Stepper Motor Holder (Autodesk Fusion 360 design; units mm, degrees)
Autodesk Fusion 360 part; units mm, degrees
note: some values were not read from the file. Set by a fixed rule: which face or edge a step refers to.
sketch "Sketch1" plane through (0, 0, 0) normal (0, 0, 1) x (1, 0, 0)
  circle A0 centre (0, 0) radius 11
  circle A1 centre (-15.5, 15.5) radius 1.5
  circle A2 centre (15.5, 15.5) radius 1.5
  circle A3 centre (15.5, -15.5) radius 1.5
  circle A4 centre (-15.5, -15.5) radius 1.5
  line L0 (23.5, -23.5) -> (-23.5, -23.5)
  line L1 (-23.5, -23.5) -> (-23.5, 23.5)
  line L2 (-23.5, 23.5) -> (23.5, 23.5)
  line L3 (23.5, 23.5) -> (23.5, -23.5)
  line L4 (23.5, -23.5) -> (-23.5, 23.5) construction
  line L5 (-23.5, -23.5) -> (23.5, 23.5) construction
  dimension "d3" = 22
  dimension "d4" = 3
  dimension "d5" = 15.5
  dimension "d6" = 15.5
  dimension "d7" = 31
  dimension "d8" = 15.5
  dimension "d9" = 47
  dimension "d10" = 47
  constraint horizontal A1.centre A2.centre
  constraint vertical A2.centre A3.centre
  constraint horizontal A3.centre A4.centre
  constraint vertical A1.centre A4.centre
  constraint equal A1 A2
  constraint equal A1 A4
  constraint equal A3 A4
  constraint coincident A0.centre origin
  constraint horizontal L0
  constraint perpendicular L0 L1
  constraint parallel L0 L2
  constraint parallel L1 L3
  constraint coincident L4 A0.centre
  constraint coincident L5 A0.centre
  measures "d3" diameter of A0
  measures "d4" diameter of A2
  measures "d5" horizontal distance of A0.centre A3.centre
  measures "d6" horizontal distance of A0.centre A4.centre
  measures "d7" distance of A1.centre A4.centre
  measures "d8" vertical distance of A0.centre A4.centre
  measures "d9" distance of L1.end L2.end
  measures "d10" distance of L0.end L1.end
extrude "Extrude1" add sketch "Sketch1" along normal blind 2
sketch "Sketch2" plane through (-23.5, 0, 0) normal (-1, 0, 0) x (0, -1, 0)
  line L0 (-23.5, 0) -> (23.5, 0)
  line L1 (23.5, 0) -> (23.5, 2)
  line L2 (23.5, 2) -> (-23.5, 2)
  line L3 (-23.5, 2) -> (-23.5, 0)
  line L4 (23.5, 2) -> (23.5, 55)
  line L5 (21, 2) -> (21, 47.4468)
  line L6 (-23.5, 2) -> (-23.5, 55)
  line L7 (-23.5, 55) -> (23.5, 55)
  line L8 (21, 47.4468) -> (21, 55)
  line L9 (23.5, 4.5) -> (-23.5, 4.5)
  line L10 (-21, 2) -> (-21, 55)
  dimension "d13" = 53
  dimension "d14" = 2.5
  dimension "d64" = 2.5
  dimension "d65" = 2.5
  dimension "d154" = 42
  constraint coincident L1.end L2.start
  constraint perpendicular L2 L4
  constraint coincident L2 L5.start
  constraint perpendicular L2 L5
  constraint coincident L2.end L3.start
  constraint perpendicular L2 L6
  constraint perpendicular L4 L7
  constraint coincident L7 L8.end
  constraint perpendicular L7 L8
  constraint coincident L4 L9.start
  constraint coincident L6 L9.end
  constraint perpendicular L6 L9
  constraint coincident L2 L10.start
  constraint coincident L7 L10.end
  constraint perpendicular L7 L10
  measures "d13" distance of L1.end L4.end
  measures "d14" distance of L4 L5
  measures "d64" distance of L2 L9
  measures "d65" distance of L6 L10
  measures "d154" distance of L5 L10
extrude "Extrude2" add sketch "Sketch2" against normal blind 2.45 contours L2 L6 L9 L10 | L2 L4 L5 L9 | L2 L5 L9 L10 | L6 L7 L9 L10 | L4 L5 L7 L8 L9 | L5 L7 L8 L9 L10
extrude "Extrude4" add sketch "Sketch2" along normal blind 2.45 from surface at -47 contours L2 L6 L9 L10 | L2 L4 L5 L9 | L2 L5 L9 L10 | L6 L7 L9 L10 | L4 L5 L7 L8 L9 | L5 L7 L8 L9 L10
extrude "Extrude5" add sketch "Sketch2" against normal up to surface (44.55 mm away) contours L2 L6 L9 L10 | L2 L4 L5 L9 | L6 L7 L9 L10 | L4 L5 L7 L8 L9
sketch "Sketch7" plane through (0, 0, 0) normal (0, 1, 0) x (1, 0, 0)
  line L0 (0, 0) -> (0, 77.058)
  circle A0 centre (0, 77.058) radius 1.1037
  dimension "d125" = 77.058
  constraint coincident L0.start origin
  constraint coincident L0.end A0.centre
  measures "d125" distance of L0.start L0.end
sketch "Sketch8" plane through (0, 21, 0) normal (0, 1, 0) x (-1, 0, 0)
  line L0 (23.5, 55) -> (-23.5, 55)
  line L1 (-23.5, 55) -> (-23.5, 0)
  line L2 (-23.5, 0) -> (23.5, 0)
  line L3 (23.5, 0) -> (23.5, 55)
  line L4 (0, 0) -> (0, 38.2341)
  circle A0 centre (-14, 40.138) radius 1.55
  circle A1 centre (14, 40.138) radius 1.55
  line L5 (11.255, 38.5532) -> (14, 36.9683)
  line L6 (14, 36.9683) -> (16.745, 38.5532)
  line L7 (16.745, 38.5532) -> (16.745, 41.7228)
  line L8 (16.745, 41.7228) -> (14, 43.3077)
  line L9 (14, 43.3077) -> (11.255, 41.7228)
  line L10 (11.255, 41.7228) -> (11.255, 38.5532)
  line L11 (-11.255, 41.7228) -> (-14, 43.3077)
  line L12 (-14, 43.3077) -> (-16.745, 41.7228)
  line L13 (-16.745, 41.7228) -> (-16.745, 38.5532)
  line L14 (-16.745, 38.5532) -> (-14, 36.9683)
  line L15 (-14, 36.9683) -> (-11.255, 38.5532)
  line L16 (-11.255, 38.5532) -> (-11.255, 41.7228)
  line L17 (21.05, 55) -> (21.05, 2)
  line L18 (21.05, 2) -> (-21.05, 2)
  line L19 (-21.05, 2) -> (-21.05, 55)
  line L20 (-21.05, 55) -> (21.05, 55)
  point P0 (14, 40.138)
  point P1 (-14, 40.138)
  dimension "d134" = 3.1
  dimension "d135" = 14
  dimension "d136" = 14
  dimension "d137" = 14.862
  dimension "d166" = 2.745
  dimension "d167" = 2.745
  constraint coincident L4.start origin
  constraint perpendicular L2 L4
  constraint horizontal P1 P0
  constraint equal A0 A1
  constraint coincident P0 A1.centre
  constraint coincident P1 A0.centre
  measures "d134" diameter of A0
  measures "d135" distance of L4 P1
  measures "d136" distance of L4 P0
  measures "d137" distance of L0 P0
  measures "d166" distance of P0 L10
  measures "d167" distance of P1 L16
extrude "Extrude8" cut sketch "Sketch8" along normal blind 2.4 contours A0 | A1 | L5 L6 L7 L8 L9 L10 | L11 L12 L13 L14 L15 L16
pattern_circular "C-Pattern2" count 4 over 360 about axis through (0, 0, 2) along (0, 0, -1) of "Extrude8"
sketch "Sketch9" plane through (0, -21, 0) normal (0, 1, 0) x (-1, 0, 0)
  line L0 (21.05, 2) -> (21.05, 55)
  line L1 (21.05, 55) -> (-21.05, 55)
  line L2 (-21.05, 55) -> (-21.05, 2)
  line L3 (-21.05, 2) -> (21.05, 2)
  line L4 (-3.75, 68) -> (3.75, 68)
  line L5 (3.75, 68) -> (3.75, 42)
  line L6 (3.75, 42) -> (-3.75, 42)
  line L7 (-3.75, 42) -> (-3.75, 68)
  line L8 (-3.75, 68) -> (3.75, 42) construction
  line L9 (3.75, 68) -> (-3.75, 42) construction
  line L10 (0, 2) -> (0, 42)
  line L11 (3.75, 42) -> (3.75, 46)
  line L12 (3.75, 46) -> (-3.75, 46)
  line L13 (-14, 43.3077) -> (-11.255, 41.7228)
  line L14 (-11.255, 41.7228) -> (-11.255, 38.5532)
  line L15 (-11.255, 38.5532) -> (-14, 36.9683)
  line L16 (-14, 36.9683) -> (-16.745, 38.5532)
  line L17 (-16.745, 38.5532) -> (-16.745, 41.7228)
  line L18 (-16.745, 41.7228) -> (-14, 43.3077)
  line L19 (14, 36.9683) -> (11.255, 38.5532)
  line L20 (11.255, 38.5532) -> (11.255, 41.7228)
  line L21 (11.255, 41.7228) -> (14, 43.3077)
  line L22 (14, 43.3077) -> (16.745, 41.7228)
  line L23 (16.745, 41.7228) -> (16.745, 38.5532)
  line L24 (16.745, 38.5532) -> (14, 36.9683)
  point P0 (0, 55)
  dimension "d143" = 7.5
  dimension "d147" = 40
  dimension "d148" = 26
  dimension "d149" = 4
  constraint horizontal L4
  constraint perpendicular L4 L5
  constraint parallel L4 L6
  constraint parallel L5 L7
  constraint coincident L8 P0
  constraint coincident L9 P0
  constraint midpoint L1 P0
  constraint midpoint L3 L10.start
  constraint perpendicular L3 L10
  constraint coincident L6 L10.end
  constraint perpendicular L6 L11
  constraint coincident L7 L12.end
  constraint perpendicular L7 L12
  measures "d143" distance of L5.end L6.end
  measures "d147" distance of L10.start L10.end
  measures "d148" distance of L4.end L5.end
  measures "d149" distance of L5.end L11.end
extrude "Extrude10" cut sketch "Sketch9" against normal blind 2 contours L5 L6 L7 L11 L12
ref_plane "WorkPlane1" through (0, 0, 39.8631) normal (0, 0, 1) x (0, 1, 0)
sketch "Sketch10" plane through (0, 0, 39.8631) normal (0, 0, 1) x (1, 0, 0)
  line L0 (-14, 23.5) -> (-17.6, 23.5)
  line L1 (-15.6, 25.5) -> (-17.6, 23.5)
  line L2 (-15.5, 23.5) -> (-15.5, 25.5)
  line L3 (-15.5, 23.5) -> (-15.5, 25.5)
  line L4 (-15.5, 25.5) -> (-15.6, 25.5)
  dimension "d156" = 3.6
  dimension "d158" = 2
  constraint perpendicular L0 L2
  constraint perpendicular L0 L3
  constraint perpendicular L3 L4
  measures "d156" distance of L0.start L0.end
  measures "d158" distance of L2.start L2.end
extrude "Extrude12" cut sketch "Sketch8" along normal blind 2.5 contours A0 | A1
sketch "Sketch11" plane through (0, 23.5, 0) normal (0, 1, 0) x (-1, 0, 0)
  circle A0 centre (14, 40.138) radius 1.55
  circle A1 centre (-14, 40.138) radius 1.55
  line L0 (23.5, 55) -> (-23.5, 55)
  line L1 (-23.5, 55) -> (-23.5, 0)
  line L2 (-23.5, 0) -> (23.5, 0)
  line L3 (23.5, 0) -> (23.5, 55)
  line L4 (23.5, 55) -> (-23.5, 55)
  line L5 (-23.5, 55) -> (-23.5, 26.165)
  line L6 (-23.5, 26.165) -> (23.5, 26.165)
  line L7 (23.5, 26.165) -> (23.5, 55)
  dimension "d170" = 28.835
  constraint horizontal L4
  constraint vertical L5
  constraint horizontal L6
  constraint vertical L7
  constraint coincident L0.start L3.end
  measures "d170" distance of L0.start L6.end
extrude "Extrude13" add sketch "Sketch11" along normal blind 1.5 contours L0 L1 L3 L4 L5 L6 L7
pattern_circular "C-Pattern4" count 4 over 360 about axis through (0, 0, 2) along (0, 0, -1) of "Extrude12", "Extrude13"
extrude "Extrude11" cut sketch "Sketch9" against normal blind 6 contours L1 L5 L7 L12
pattern_circular "C-Pattern5" count 4 over 360 about axis through (0, 0, 2) along (0, 0, -1) of "Extrude10", "Extrude11"
extrude "Extrude14" add 2 faces at (-24, 23.5, 45.3883) (24, 23.5, 35.7767) along direction (0, 1, 0) blind 1.5
extrude "Extrude15" add 2 faces at (24.5, -23.5, 35.7767) (-24, -23.5, 35.7767) along direction (0, -1, 0) blind 1.5
fillet "Fillet2" radius 5 4 edges at (25, 25, 40.5825) (-25, 25, 40.5825) (25, -25, 40.5825) (-25, -25, 40.5825)
chamfer "Chamfer2" distance 1.5 angle 45 12 edges at (23.5, -23.5, 13.0825) (23.5, 23.5, 13.0825) (-23.5, 23.5, 13.0825) (-23.5, -23.5, 13.0825) (-25, 0, 26.165) (-23.5355, 23.5355, 26.165) (0, 25, 26.165) (23.5355, 23.5355, 26.165) (25, 0, 26.165) (23.5355, -23.5355, 26.165) (0, -25, 26.165) (-23.5355, -23.5355, 26.165)
extrude "Extrude16" cut 1 faces at (0.274, 14.7716, 2) along direction (0, 0, -1) blind 0.2
sketch "Sketch13" plane through (0, 25, 0) normal (0, 1, 0) x (-1, 0, 0)
  circle A0 centre (-14, 40.138) radius 1.55
  circle A1 centre (14, 40.138) radius 1.55
  line L0 (-20, 27.665) -> (20, 27.665)
  line L1 (20, 27.665) -> (20, 55)
  line L2 (20, 55) -> (3.75, 55)
  line L3 (3.75, 55) -> (3.75, 46)
  line L4 (3.75, 46) -> (-3.75, 46)
  line L5 (-3.75, 46) -> (-3.75, 55)
  line L6 (-3.75, 55) -> (-20, 55)
  line L7 (-20, 55) -> (-20, 27.665)
  circle A2 centre (-14, 40.138) radius 1.55
  circle A3 centre (14, 40.138) radius 1.55
equation "d5 = ( 31 / 2 ) * 1 mm"
equation "d125 = 49.5 mm + ( 55.116 / 2 ) * 1 mm"
equation "d135 = 12.5 mm + 1.5 mm"
equation "d137 = 13.312 mm + ( ( 3.1 / 2 ) * 1 mm )"
equation "d170 = 27.335 mm + 1.5 mm"
